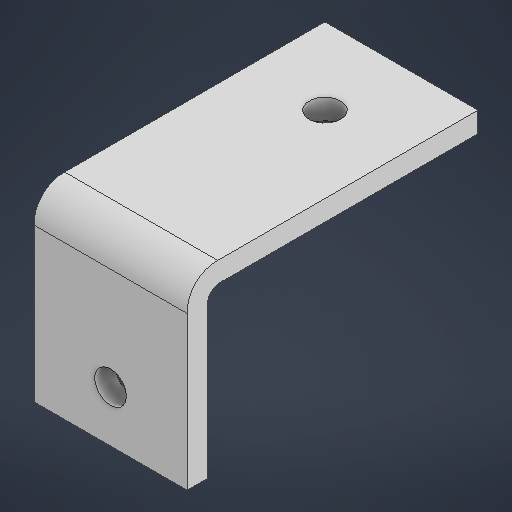
# Autodesk Inventor part: Slider Holding Bracket
Saved by Autodesk Inventor 2027 (Build 310192000, 192)
## iProperties
Created: 2026-04-16
Part Number: Slider Holding Bracket
Material: Generic
Document SubType Name: Modeling
Designer: ratik
Density: 1 g/cm^3
Appearance: Default
Author: ratik
Autodesk Inventor part; units mm, degrees
ref_plane "YZ Plane" through (0, 0, 0) normal (1, 0, 0) x (0, 1, 0)
ref_plane "XZ Plane" through (0, 0, 0) normal (0, 1, 0) x (-1, 0, 0)
ref_plane "XY Plane" through (0, 0, 0) normal (0, 0, 1) x (1, 0, 0)
sketch "Sketch1" plane through (0, 0, 0) normal (1, 0, 0) x (0, 1, 0)
  line L0 (-11.8519, 0.5556) -> (-11.8519, -49.4444)
  line L1 (-11.8519, -49.4444) -> (-7.8519, -49.4444)
  line L2 (-7.8519, -49.4444) -> (-7.8519, 1.5556)
  line L3 (-13.8519, 7.5556) -> (-43.8519, 7.5556)
  line L4 (-43.8519, 7.5556) -> (-43.8519, 3.5556)
  line L5 (-43.8519, 3.5556) -> (-13.8519, 3.5556)
  arc A0 (-7.8519, 1.5556) -> (-13.8519, 7.5556) centre (-13.5586, 1.8488) ccw
  arc A1 (-11.8519, 0.5556) -> (-13.8519, 3.5556) centre (-14.3519, 1.0556) ccw
  point P0 (0, 0)
  dimension "d0" = 4
  dimension "d1" = 4
  dimension "d2" = 50
  dimension "d3" = 57
  dimension "d4" = 30
  dimension "d18" = 30
  constraints: 12 end point, 4 point on circle, 2 centre point, 2 parallel, 1 horizontal, 1 perpendicular
  measures "d0" distance of L0.end L1.end
  measures "d1" distance of L3.end L4.end
  measures "d2" distance of L0.start L0.end
  measures "d3" distance between parallel lines of L1 L3
  measures "d4" distance of L3.start L3.end
  measures "d18" distance of L4.end L5.end
extrude "Extrusion1" add sketch "Sketch1" along normal blind 30
sketch "Sketch2" plane through (0, -7.8519, 1.5556) normal (0, 1, 0) x (1, 0, 0)
  circle A0 centre (15, 36) radius 3.1
  line L0 (30, 51) -> (30, 0) projected
  line L1 (0, -6) -> (30, -6) projected
  point P0 (0, 1.5556)
  dimension "d8" = 6.2
  dimension "d9" = 15
  dimension "d10" = 42
  constraints: 1 centre point
  measures "d8" diameter of A0
  measures "d9" distance from line of L0 A0.centre
  measures "d10" distance from line of L1 A0.centre
extrude "Extrusion2" cut sketch "Sketch2" against normal blind 30
sketch "Sketch3" plane through (0, -43.8519, 7.5556) normal (0, 0, 1) x (1, 0, 0)
  circle A0 centre (15, 10) radius 3.1
  line L0 (30, 30) -> (30, 0) projected
  line L1 (0, 0) -> (30, 0) projected
  point P0 (0, 43.8519)
  dimension "d13" = 6.2
  dimension "d14" = 15
  dimension "d15" = 10
  constraints: 1 centre point
  measures "d13" diameter of A0
  measures "d14" distance from line of L0 A0.centre
  measures "d15" distance from line of L1 A0.centre
extrude "Extrusion3" cut sketch "Sketch3" against normal blind 30
body "Solid1"
